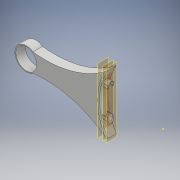
# Autodesk Inventor part: Aile
Saved by Autodesk Inventor 2017 (Build 210142000, 142)
## iProperties
Part Number: Aile
Material: Générique
Document SubType Name: Modeling
Designer: Thomas
Density: 1 g/cm^3
Appearance: Par défaut
Author: Thomas
Autodesk Inventor part; units mm, degrees
ref_plane "YZ Plane" through (0, 0, 0) normal (1, 0, 0) x (0, 1, 0)
ref_plane "XZ Plane" through (0, 0, 0) normal (0, 1, 0) x (-1, 0, 0)
ref_plane "XY Plane" through (0, 0, 0) normal (0, 0, 1) x (1, 0, 0)
sketch "Esquisse1" plane through (0, 0, 0) normal (0, 1, 0) x (-1, 0, 0)
  arc A0 (51.3642, -31.0232) -> (51.3642, 31) centre (0, -0.0116) ccw
  arc A1 (129, -9.7584) -> (129, 9.7352) centre (136, -0.0116) ccw
  arc A2 (51.3642, 31) -> (129, 9.7352) centre (116, 114.6263) ccw
  line L0 (64, -0.0116) -> (129, -0.0116) construction
  arc A3 (129, -9.7584) -> (129, 9.7352) centre (136, -0.0116) ccw
  arc A4 (129, -9.7584) -> (51.3642, -31.0232) centre (116, -114.6495) ccw
  circle A5 centre (136, -0.0116) radius 11
  point P0 (0, 0)
  dimension "d0" = 120
  dimension "d1" = 24
  dimension "d2" = 22
  constraints: 10 point on circle, 6 centre point, 3 symmetric about line, 2 end point, 1 coincident, 1 horizontal, 2 other
  measures "d0" diameter of A0
  measures "d1" diameter of A1
  measures "d2" diameter of A5
extrude "Extrusion1" add sketch "Esquisse1" along normal blind 10
ref_plane "Plan de construction1" through (-51.3642, 0, -31.0232) normal (1, 0, 0) x (0, 1, 0)
sketch "Esquisse2" plane through (-51.3642, 0, -31.0232) normal (1, 0, 0) x (0, 1, 0)
  line L0 (5, 64.5652) -> (5, -0.1304) construction
  line L1 (3, 49) -> (7, 49)
  line L2 (8, 47.6173) -> (8, 44)
  line L3 (2, 44) -> (2, 47.6173)
  line L4 (2, 49) -> (8, 43) construction
  line L5 (8, 49) -> (2, 43) construction
  line L6 (8, 18) -> (8, 14.5151)
  line L7 (7, 13) -> (3, 13)
  line L8 (2, 14.5151) -> (2, 18)
  line L9 (2, 19) -> (8, 13) construction
  line L10 (8, 19) -> (2, 13) construction
  line L11 (10, 62.0232) -> (10, 0) projected
  line L12 (0, 0) -> (10, 0) projected
  line L13 (0, 62.0232) -> (10, 62.0232) projected
  spline S0 degree 4 poles (7.6671, 44) (6.4354, 47.4326) (4.9707, 48.7302) (3.6119, 47.2748) (2.3584, 44) knots 0 0 0 0 0 1 1 1 1 1
  spline S1 degree 4 poles (7.6511, 18) (6.3929, 14.6165) (5, 13.0055) (3.6071, 14.6165) (2.3489, 18) knots 0 0 0 0 0 1 1 1 1 1
  arc A0 (8, 47.4506) -> (7, 49) centre (6.4288, 47.5339) ccw
  arc A1 (3, 49) -> (2, 47.4506) centre (3.5712, 47.5339) ccw
  arc A2 (7, 13) -> (8, 14.5151) centre (6.3523, 14.5151) ccw
  arc A3 (2, 14.5151) -> (3, 13) centre (3.6477, 14.5151) ccw
  line L14 (2, 18) -> (2.3489, 18)
  line L15 (7.6511, 18) -> (8, 18)
  line L16 (2.776, 16.8516) -> (1.9218, 19.1484) construction
  arc A4 (2.0268, 18.9251) -> (2.7095, 17.0892) centre (24.2353, 26.1386) ccw construction
  line L17 (8.0782, 19.1484) -> (7.224, 16.8516) construction
  arc A5 (7.2905, 17.0892) -> (7.9732, 18.9251) centre (-14.2353, 26.1386) ccw construction
  line L18 (2, 44) -> (2.3584, 44)
  line L19 (7.6671, 44) -> (8, 44)
  line L20 (2.7888, 45.1243) -> (1.9281, 42.8757) construction
  arc A6 (2.7221, 44.891) -> (2.0343, 43.0939) centre (22.8073, 36.1728) ccw construction
  line L21 (8.0877, 42.828) -> (7.2466, 45.172) construction
  arc A7 (7.9784, 43.0548) -> (7.3065, 44.9274) centre (-10.0817, 37.6313) ccw construction
  point P0 (0, 31.0232)
  point P1 (5, 46)
  point P2 (5, 16)
  dimension "d10" = 2
  dimension "d11" = 2
  dimension "d12" = 13
  dimension "d13" = 13.0232
  dimension "d19" = 1
  dimension "d20" = 1
  dimension "d21" = 1
  dimension "d22" = 1
  constraints: 38 end point, 14 point on circle, 12 midpoint, 8 centre point, 8 point on line, 6 symmetric about line, 3 perpendicular, 2 parallel, 1 horizontal, 1 tangent, 1 vertical, 16 other
  measures "d10" distance between parallel lines of L11 L6
  measures "d11" distance between parallel lines of L11 L2
  measures "d12" distance between parallel lines of L12 L7
  measures "d13" distance between parallel lines of L13 L1
  measures "d19" distance from line of L10.start L15
  measures "d20" distance from line of L9.start L14
  measures "d21" distance from line of L5.end L18
  measures "d22" distance from line of L4.end L19
extrude "Extrusion2" add sketch "Esquisse2" against normal blind 10
sketch "Esquisse3" plane through (-51.3642, 8, 16.594) normal (0, 1, 0) x (1, 0, 0)
  point P0 (51.3642, 16.594)
sketch "Esquisse4" plane through (-51.3642, 8, 16.594) normal (0, 1, 0) x (1, 0, 0)
  point P0 (51.3642, 16.594)
ref_plane "Plan de construction7" through (-55.0062, 0, -31.0232) normal (1, 0, 0) x (0, 1, 0)
ref_plane "Plan de construction6" through (-60.1142, 0, -31.0232) normal (1, 0, 0) x (0, 1, 0)
fillet "Congé2" radius 1 1 edges at (-60, 0, -0.0116)
sketch "Esquisse7" plane through (-51.3642, 0, -31.0232) normal (1, 0, 0) x (0, 1, 0)
  line L0 (7, 49) -> (3, 49) projected
  line L1 (4, 49) -> (6, 49)
  line L2 (6, 49) -> (6, 50)
  line L3 (6, 50) -> (4, 50)
  line L4 (4, 50) -> (4, 49)
  line L5 (3, 13) -> (7, 13) projected
  line L6 (4, 13) -> (6, 13)
  line L7 (6, 13) -> (6, 12)
  line L8 (6, 12) -> (4, 12)
  line L9 (4, 12) -> (4, 13)
  point P0 (0, 31.0232)
  constraints: 16 end point, 4 parallel, 3 point on line, 2 horizontal, 2 perpendicular
extrude "Extrusion5" add sketch "Esquisse7" against normal blind 1
ref_plane "Plan de construction8" through (-51.3642, 4, -19.0232) normal (0, -1, 0) x (1, 0, 0)
sketch "Esquisse8" plane through (-51.3642, 4, -19.0232) normal (0, -1, 0) x (1, 0, 0)
  line L0 (-1, 37) -> (-1, 38) projected
  line L1 (0, 37) -> (-1, 37) projected
  line L2 (0, 1) -> (0, 0) projected
  line L3 (-1, 1) -> (-1, 0)
  line L4 (0, 1) -> (-5.8685, 1) projected
  line L5 (0, 38) -> (-1, 38) projected
  line L6 (-1, 37) -> (-1, 38)
  line L7 (-1, 0) -> (-1, 1) projected
  line L8 (0, 0) -> (0, 1) projected
  line L9 (-1, 1) -> (0, 1) projected
  line L10 (-1, 0) -> (-1, 1) projected
  line L11 (0, 0) -> (-1, 0) projected
  line L12 (0, 0) -> (0, 1) projected
  line L13 (-1, 1) -> (0, 1) projected
  line L14 (-1, 0) -> (-1, 1) projected
  line L15 (0, 0) -> (-1, 0) projected
  line L16 (0, 38) -> (0, 37) projected
  line L17 (0, 38) -> (-1, 38) projected
  line L18 (-1, 37) -> (-1, 38) projected
  line L19 (0, 37) -> (-1, 37) projected
  line L20 (0, 0) -> (-1, 0) projected
  line L21 (0, 1) -> (-1, 1) projected
  arc A0 (-0.1986, 0) -> (-1, 1) centre (-1.3637, -0.1126) ccw
  line L22 (0, 38) -> (-1, 38) projected
  arc A1 (-1, 37) -> (-0.1986, 38) centre (-1.3356, 38.0901) ccw
  point P0 (51.3642, 19.0232)
  constraints: 4 end point, 4 point on circle, 2 centre point, 2 point on line, 1 collinear, 1 perpendicular
extrude "Extrusion6" cut sketch "Esquisse8" against normal blind 3.25 contours L0 L5 A1 | A0 L11 L3
sketch "Esquisse9" plane through (0, 0, 0) normal (0, 1, 0) x (-1, 0, 0)
  line L0 (51.3642, 17.9768) -> (57.24, 17.9768) projected
  circle A0 centre (0, 0) radius 54.4192
  constraints: 1 coincident, 3 other
extrude "Extrusion7" cut sketch "Esquisse9" along normal blind 10.25
